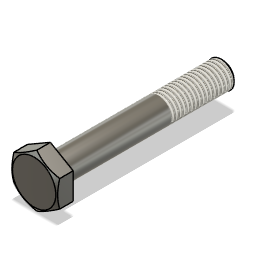
body part (v2~recovered) (Autodesk Fusion 360 archive; units mm, degrees)
design "Heavy Hex Screw ANSI B18.2.3.3M - M14x2 x 90 Steel Grade 2 Plain"
description: Heavy Hex Screw ANSI B18.2.3.3M - M14x2 x 90
Autodesk Fusion 360 part; units mm, degrees
sketch "Sketch1" plane through (0, 0, 0) normal (0, 1, 0) x (1, 0, 0)
  line L0 (-7, 0) -> (-7, 90)
  line L1 (-7, 90) -> (0, 90)
  line L2 (0, 90) -> (0, -9.09)
  line L3 (-11.25, -0.6) -> (-13.86, -0.6)
  line L4 (-13.86, -0.6) -> (-13.86, -7.6697)
  line L5 (-11.25, -0.6) -> (-10.9036, 0)
  line L6 (-10.9036, 0) -> (-7, 0)
  line L7 (0, -9.09) -> (-11.4, -9.09)
  line L8 (-13.86, -7.6697) -> (-11.4, -9.09)
  dimension "d81" = 27.72
  dimension "d123" = 0.6
  dimension "d127" = 90
  dimension "d149" = 14
  dimension "d157" = 30
  dimension "d158" = 22.8
  dimension "d162" = 9.09
  dimension "d163" = 30
  dimension "d164" = 22.5
  constraint perpendicular L0 L1
  constraint perpendicular L0 L3
  constraint vertical L0
  constraint vertical L2
  constraint parallel L2 L4
  constraint coincident L2 L7.start
  constraint perpendicular L0 L6
  constraint coincident origin L6
  constraint coincident L0.end L1.start
  constraint perpendicular L2 L7
  constraint coincident origin L2
  measures "d123" distance of L3 L6
  measures "d127" distance of L1 L6
  measures "d157" angle of L7 L8
  measures "d162" distance of L6 L7
  measures "d163" angle of L4 L5
revolve "Revolve1" add sketch "Sketch1" angle 360 about axis through (0, 0, -90) along (0, 0, 1)
sketch "Sketch8" plane through (0, 0, 0) normal (0, 0, 1) x (1, 0, 0)
  line L0 (-12, -6.9354) -> (-12, 6.9354)
  circle A0 centre (0, 0) radius 10.45
  circle A1 centre (0, 0) radius 13.86
  circle A2 centre (0, 0) radius 13.86
  dimension "d114" = 12
  constraint vertical L0
  constraint coincident L0.end A1
  constraint coincident L0.start A2
  measures "d114" distance of A0.centre L0
extrude "Extrude5" cut sketch "Sketch8" along normal through all contours L0 A1 A2 picked at (-12.3001, -1.6893)
pattern_circular "C-Pattern2" count 6 over 360 about axis through (0, 0, 1.75) along (0, 0, 1) of "Extrude5"
thread "Thread2" "ISO Metric profile 14.0 M14x2 6g" major diameter 13.822 minor diameter 11.534 pitch 2 angle 60 resizes the face on face at (-6.9652, 0.697, -60) from (0, 0, -56) to (0, 0, -90)
fillet "Fillet6" radius 0.6 1 edges at (6.911, 0, 0)
sketch "Sketch15" plane through (0, 0, 0) normal (0, 1, 0) x (1, 0, 0)
  line L0 (-7.14, 90) -> (-7.14, 88.7731)
  line L1 (-7.14, 88.7731) -> (-5.7731, 90)
  line L2 (0, 90) -> (0, -9.09)
  line L3 (-7.14, 90) -> (0, 90)
  dimension "d152" = 7.14
  dimension "d153" = 5.7731
  dimension "d154" = 1.2269
  constraint coincident L2.start L3.end
  constraint perpendicular L2 L3
  constraint coincident L1.end L3
  constraint perpendicular L0 L3
  measures "d152" horizontal distance of origin L0.start
  measures "d153" horizontal distance of origin L1.end
  measures "d154" distance of L0.start L0.end
revolve "Revolve4" cut sketch "Sketch15" angle 360 about axis through (0, 0, 1.75) along (0, 0, 1)
equation "adsk_nomlen = 90.00 mm"
equation "adsk_headh = 9.09 mm"
equation "adsk_headdia = 27.72 mm"
equation "adsk_nomdia = 14.00 mm"
equation "d81 = adsk_headdia"
equation "adsk_waflat = 24.00 mm"
equation "d114 = adsk_waflat / 2"
equation "adsk_thrlen = 34.00 mm"
equation "adsk_chamang2 = 30.00 deg"
equation "adsk_midfillet = 0.60 mm"
equation "d123 = adsk_necklen"
equation "adsk_necklen = 0.60 mm"
equation "adsk_neckdia = 22.50 mm"
equation "d127 = adsk_nomlen"
equation "d138 = adsk_midfillet"
equation "d140 = min(adsk_thrlen; adsk_nomlen - adsk_midfillet - 0.01 mm)"
equation "adsk_endpointdia = 11.5462 mm"
equation "adsk_startlen = 1.2269 mm"
equation "d149 = adsk_nomdia"
equation "d152 = adsk_nomdia * 0.51"
equation "d153 = adsk_endpointdia / 2"
equation "d154 = adsk_startlen"
equation "d157 = adsk_chamang2"
equation "d158 = adsk_waflat * 0.95"
equation "adsk_neckang = 30 deg"
equation "d162 = adsk_headh"
equation "d163 = adsk_neckang"
equation "d164 = adsk_neckdia"

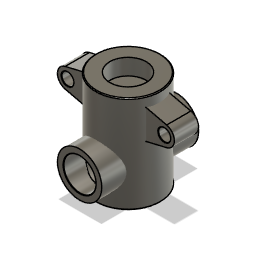
design "wheel hub"
Autodesk Fusion 360 part; units mm, degrees
sketch "Sketch1" plane through (0, 0, 0) normal (0, 0, 1) x (1, 0, 0)
  line L0 (0, 0) -> (40, 0)
  line L1 (40, 0) -> (40, 120)
  line L2 (40, 120) -> (0, 120)
  line L3 (0, 120) -> (0, 0)
  dimension "d1" = 40
  dimension "d2" = 120
  constraint horizontal L0
  constraint vertical L1
  constraint horizontal L2
  constraint vertical L3
  constraint coincident L0.start L3.end
  measures "d1" distance of L1.end L2.end
  measures "d2" distance of L0.end L1.end
revolve "Revolve1" add sketch "Sketch1" angle 360 about axis through (0, 120, 0) along (0, -1, 0) makes body 1
sketch "Sketch2" plane through (0, 0, 0) normal (0, 0, 1) x (1, 0, 0)
sketch "Sketch3" plane through (0, 0, 0) normal (0, 0, 1) x (1, 0, 0)
  line L0 (0, 150) -> (0, -10) construction
  line L1 (-70, 90) -> (60, 90) construction
  line L2 (30, 110) -> (30, 70)
  line L3 (30, 70) -> (62.898, 77.8406)
  line L4 (30, 110) -> (62.898, 102.1594)
  circle A0 centre (60, 90) radius 7.5
  arc A1 (62.898, 77.8406) -> (62.898, 102.1594) centre (60, 90) ccw
  point P0 (40, 120)
  dimension "d4" = 25
  dimension "d5" = 20
  dimension "d6" = 40
  dimension "d7" = 10
  dimension "d8" = 15
  constraint vertical L0
  constraint perpendicular L0 L1
  constraint coincident L1.end A0.centre
  constraint perpendicular L1 L2
  constraint tangent L4 A1
  constraint tangent L3 A1
  constraint concentric A0 A1
  measures "d4" diameter of A1
  measures "d5" distance of L1 L2.start
  measures "d6" distance of L2.start L2.end
  measures "d7" horizontal distance of L2.start P0
  measures "d8" diameter of A0
extrude "Extrude1" add sketch "Sketch3" along normal blind 15 and the other way blind 15 separate body makes body 2
sketch "Sketch4" plane through (0, 0, 0) normal (0, 0, 1) x (1, 0, 0)
mirror "Mirror1" about plane through (0, 0, 0) normal (1, 0, 0) of bodies 2 makes body 3
sketch "Sketch5" plane through (0, 0, 0) normal (0, 0, 1) x (1, 0, 0)
  circle A0 centre (0, 40) radius 27.5
  line L0 (-40, 0) -> (40, 0)
  dimension "d15" = 55
  dimension "d16" = 40
  measures "d15" diameter of A0
  measures "d16" distance of A0.centre L0
extrude "Extrude2" add sketch "Sketch5" along normal blind 60 and the other way blind 60 separate body makes body 4
sketch "Sketch6" plane through (0, 0, 60) normal (0, 0, 1) x (1, 0, 0)
  circle A0 centre (0, 40) radius 27.5
  circle A1 centre (0, 40) radius 20
  dimension "d21" = 40
  constraint concentric A0 A1
  measures "d21" diameter of A1
extrude "Extrude3" cut sketch "Sketch6" along normal blind 60 and the other way blind 60 contours A1 bodies 1 4
sketch "Sketch7" plane through (0, 120, 0) normal (0, 1, 0) x (-1, 0, 0)
  circle A0 centre (0, 0) radius 40
  circle A1 centre (0, 0) radius 22.5
  dimension "d26" = 45
  constraint concentric A0 A1
  measures "d26" diameter of A1
extrude "Extrude4" cut 4 faces at (-6.8687, 44.386, 0) (-6.8687, 44.386, 0) (-6.8687, 44.386, 0) (-6.8687, 44.386, 0) along direction (0, 0, 1) blind 60 and the other way blind 60 on bodies 1 4 bodies 1 4
extrude "Extrude5" cut sketch "Sketch7" along normal blind 0 and the other way blind 20 contours A1 bodies 1
fillet "Fillet1" radius 1 12 edges at (20, 40, 34.641) (20, 40, -34.641) (-37.2931, 0, -14.4646) (-37.2931, 120, -14.4646) (30, 90, 15) (30, 110, 0) (30, 90, -15) (30, 70, 0) (-30, 90, 15) (-30, 110, 0) (-30, 90, -15) (-30, 70, 0) 1 faces at (23.3497, 53.3659, 32.4776) on bodies 1 2 3
chamfer "Chamfer1" distance 0.5 angle 45 6 edges at (53.0075, 92.7121, 15) (53.0075, 87.2879, -15) (-53.0075, 92.7121, 15) (-53.0075, 87.2879, -15) (-18.6465, 47.2323, 60) (-18.6465, 32.7677, -60) measured on face at (38.3212, 90, 15) measured on face at (38.3212, 90, -15) measured on face at (-67.4627, 89.2532, 5) measured on face at (-67.4627, 89.2532, 5) measured on face at (24.8232, 37.6402, 60) measured on face at (24.8232, 37.6402, -60) on bodies 2 3 4

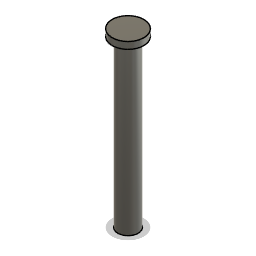
design "landing gear piston"
Autodesk Fusion 360 part; units mm, degrees
sketch "Sketch1" plane through (0, 0, 0) normal (0, 0, 1) x (1, 0, 0)
  line L0 (0, 0) -> (0, 380)
  line L1 (0, 380) -> (35, 380)
  line L2 (35, 380) -> (35, 365)
  line L3 (35, 365) -> (22.5, 365)
  line L4 (22.5, 365) -> (22.5, 0)
  line L5 (22.5, 0) -> (0, 0)
  dimension "d2" = 380
  dimension "d3" = 22.5
  dimension "d4" = 35
  dimension "d5" = 15
  constraint coincident L0.start L5.end
  constraint perpendicular L1 L2
  constraint perpendicular L3 L4
  constraint perpendicular L0 L5
  measures "d2" distance of L0.start L0.end
  measures "d3" distance of L4.end L0.start
  measures "d4" distance of L0.end L1.end
  measures "d5" distance of L1.end L2.end
revolve "Revolve1" add sketch "Sketch1" angle 360 about axis through (0, 0, 0) along (0, 1, 0)

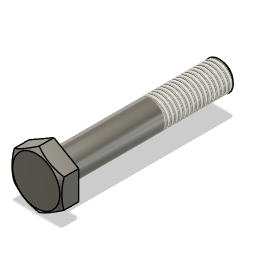
design "Heavy Hex Screw ANSI B18.2.3.3M - M14x2 x 80 Steel Grade 2 Plain"
description: Heavy Hex Screw ANSI B18.2.3.3M - M14x2 x 80
Autodesk Fusion 360 part; units mm, degrees
sketch "Sketch1" plane through (0, 0, 0) normal (0, 1, 0) x (1, 0, 0)
  line L0 (-7, 0) -> (-7, 80)
  line L1 (-7, 80) -> (0, 80)
  line L2 (0, 80) -> (0, -9.09)
  line L3 (-11.25, -0.6) -> (-13.86, -0.6)
  line L4 (-13.86, -0.6) -> (-13.86, -7.6697)
  line L5 (-11.25, -0.6) -> (-10.9036, 0)
  line L6 (-10.9036, 0) -> (-7, 0)
  line L7 (0, -9.09) -> (-11.4, -9.09)
  line L8 (-13.86, -7.6697) -> (-11.4, -9.09)
  dimension "d81" = 27.72
  dimension "d123" = 0.6
  dimension "d127" = 80
  dimension "d149" = 14
  dimension "d157" = 30
  dimension "d158" = 22.8
  dimension "d162" = 9.09
  dimension "d163" = 30
  dimension "d164" = 22.5
  constraint perpendicular L0 L1
  constraint perpendicular L0 L3
  constraint vertical L0
  constraint vertical L2
  constraint parallel L2 L4
  constraint coincident L2 L7.start
  constraint perpendicular L0 L6
  constraint coincident origin L6
  constraint coincident L0.end L1.start
  constraint perpendicular L2 L7
  constraint coincident origin L2
  measures "d123" distance of L3 L6
  measures "d127" distance of L1 L6
  measures "d157" angle of L7 L8
  measures "d162" distance of L6 L7
  measures "d163" angle of L4 L5
revolve "Revolve1" add sketch "Sketch1" angle 360 about axis through (0, 0, -80) along (0, 0, 1)
sketch "Sketch8" plane through (0, 0, 0) normal (0, 0, 1) x (1, 0, 0)
  line L0 (-12, -6.9354) -> (-12, 6.9354)
  circle A0 centre (0, 0) radius 10.45
  circle A1 centre (0, 0) radius 13.86
  circle A2 centre (0, 0) radius 13.86
  dimension "d114" = 12
  constraint vertical L0
  constraint coincident L0.end A1
  constraint coincident L0.start A2
  measures "d114" distance of A0.centre L0
extrude "Extrude5" cut sketch "Sketch8" along normal through all contours L0 A1 A2 picked at (-12.3001, -1.6893)
pattern_circular "C-Pattern2" count 6 over 360 about axis through (0, 0, 1.75) along (0, 0, 1) of "Extrude5"
thread "Thread2" "ISO Metric profile 14.0 M14x2 6g" major diameter 13.822 minor diameter 11.534 pitch 2 angle 60 resizes the face on face at (-6.9913, 0.3489, -53.3333) from (0, 0, -46) to (0, 0, -80)
fillet "Fillet6" radius 0.6 1 edges at (6.911, 0, 0)
sketch "Sketch15" plane through (0, 0, 0) normal (0, 1, 0) x (1, 0, 0)
  line L0 (-7.14, 80) -> (-7.14, 78.7731)
  line L1 (-7.14, 78.7731) -> (-5.7731, 80)
  line L2 (0, 80) -> (0, -9.09)
  line L3 (-7.14, 80) -> (0, 80)
  dimension "d152" = 7.14
  dimension "d153" = 5.7731
  dimension "d154" = 1.2269
  constraint coincident L2.start L3.end
  constraint perpendicular L2 L3
  constraint coincident L1.end L3
  constraint perpendicular L0 L3
  measures "d152" horizontal distance of origin L0.start
  measures "d153" horizontal distance of origin L1.end
  measures "d154" distance of L0.start L0.end
revolve "Revolve4" cut sketch "Sketch15" angle 360 about axis through (0, 0, 1.75) along (0, 0, 1)
equation "adsk_nomlen = 80.00 mm"
equation "adsk_headh = 9.09 mm"
equation "adsk_headdia = 27.72 mm"
equation "adsk_nomdia = 14.00 mm"
equation "d81 = adsk_headdia"
equation "adsk_waflat = 24.00 mm"
equation "d114 = adsk_waflat / 2"
equation "adsk_thrlen = 34.00 mm"
equation "adsk_chamang2 = 30.00 deg"
equation "adsk_midfillet = 0.60 mm"
equation "d123 = adsk_necklen"
equation "adsk_necklen = 0.60 mm"
equation "adsk_neckdia = 22.50 mm"
equation "d127 = adsk_nomlen"
equation "d138 = adsk_midfillet"
equation "d140 = min(adsk_thrlen; adsk_nomlen - adsk_midfillet - 0.01 mm)"
equation "adsk_endpointdia = 11.5462 mm"
equation "adsk_startlen = 1.2269 mm"
equation "d149 = adsk_nomdia"
equation "d152 = adsk_nomdia * 0.51"
equation "d153 = adsk_endpointdia / 2"
equation "d154 = adsk_startlen"
equation "d157 = adsk_chamang2"
equation "d158 = adsk_waflat * 0.95"
equation "adsk_neckang = 30 deg"
equation "d162 = adsk_headh"
equation "d163 = adsk_neckang"
equation "d164 = adsk_neckdia"

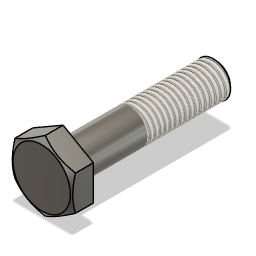
design "Heavy Hex Screw ANSI B18.2.3.3M - M14x2 x 60 Steel Grade 2 Plain"
description: Heavy Hex Screw ANSI B18.2.3.3M - M14x2 x 60
Autodesk Fusion 360 part; units mm, degrees
sketch "Sketch1" plane through (0, 0, 0) normal (0, 1, 0) x (1, 0, 0)
  line L0 (-7, 0) -> (-7, 60)
  line L1 (-7, 60) -> (0, 60)
  line L2 (0, 60) -> (0, -9.09)
  line L3 (-11.25, -0.6) -> (-13.86, -0.6)
  line L4 (-13.86, -0.6) -> (-13.86, -7.6697)
  line L5 (-11.25, -0.6) -> (-10.9036, 0)
  line L6 (-10.9036, 0) -> (-7, 0)
  line L7 (0, -9.09) -> (-11.4, -9.09)
  line L8 (-13.86, -7.6697) -> (-11.4, -9.09)
  dimension "d81" = 27.72
  dimension "d123" = 0.6
  dimension "d127" = 60
  dimension "d149" = 14
  dimension "d157" = 30
  dimension "d158" = 22.8
  dimension "d162" = 9.09
  dimension "d163" = 30
  dimension "d164" = 22.5
  constraint perpendicular L0 L1
  constraint perpendicular L0 L3
  constraint vertical L0
  constraint vertical L2
  constraint parallel L2 L4
  constraint coincident L2 L7.start
  constraint perpendicular L0 L6
  constraint coincident origin L6
  constraint coincident L0.end L1.start
  constraint perpendicular L2 L7
  constraint coincident origin L2
  measures "d123" distance of L3 L6
  measures "d127" distance of L1 L6
  measures "d157" angle of L7 L8
  measures "d162" distance of L6 L7
  measures "d163" angle of L4 L5
revolve "Revolve1" add sketch "Sketch1" angle 360 about axis through (0, 0, -60) along (0, 0, 1)
sketch "Sketch8" plane through (0, 0, 0) normal (0, 0, 1) x (1, 0, 0)
  line L0 (-12, -6.9354) -> (-12, 6.9354)
  circle A0 centre (0, 0) radius 10.45
  circle A1 centre (0, 0) radius 13.86
  circle A2 centre (0, 0) radius 13.86
  dimension "d114" = 12
  constraint vertical L0
  constraint coincident L0.end A1
  constraint coincident L0.start A2
  measures "d114" distance of A0.centre L0
extrude "Extrude5" cut sketch "Sketch8" along normal through all contours L0 A1 A2 picked at (-12.3001, -1.6893)
pattern_circular "C-Pattern2" count 6 over 360 about axis through (0, 0, 1.75) along (0, 0, 1) of "Extrude5"
thread "Thread2" "ISO Metric profile 14.0 M14x2 6g" major diameter 13.822 minor diameter 11.534 pitch 2 angle 60 resizes the face on face at (-6.9652, 0.697, -40) from (0, 0, -26) to (0, 0, -60)
fillet "Fillet6" radius 0.6 1 edges at (6.911, 0, 0)
sketch "Sketch15" plane through (0, 0, 0) normal (0, 1, 0) x (1, 0, 0)
  line L0 (-7.14, 60) -> (-7.14, 58.7731)
  line L1 (-7.14, 58.7731) -> (-5.7731, 60)
  line L2 (0, 60) -> (0, -9.09)
  line L3 (-7.14, 60) -> (0, 60)
  dimension "d152" = 7.14
  dimension "d153" = 5.7731
  dimension "d154" = 1.2269
  constraint coincident L2.start L3.end
  constraint perpendicular L2 L3
  constraint coincident L1.end L3
  constraint perpendicular L0 L3
  measures "d152" horizontal distance of origin L0.start
  measures "d153" horizontal distance of origin L1.end
  measures "d154" distance of L0.start L0.end
revolve "Revolve4" cut sketch "Sketch15" angle 360 about axis through (0, 0, 1.75) along (0, 0, 1)
equation "adsk_nomlen = 60.00 mm"
equation "adsk_headh = 9.09 mm"
equation "adsk_headdia = 27.72 mm"
equation "adsk_nomdia = 14.00 mm"
equation "d81 = adsk_headdia"
equation "adsk_waflat = 24.00 mm"
equation "d114 = adsk_waflat / 2"
equation "adsk_thrlen = 34.00 mm"
equation "adsk_chamang2 = 30.00 deg"
equation "adsk_midfillet = 0.60 mm"
equation "d123 = adsk_necklen"
equation "adsk_necklen = 0.60 mm"
equation "adsk_neckdia = 22.50 mm"
equation "d127 = adsk_nomlen"
equation "d138 = adsk_midfillet"
equation "d140 = min(adsk_thrlen; adsk_nomlen - adsk_midfillet - 0.01 mm)"
equation "adsk_endpointdia = 11.5462 mm"
equation "adsk_startlen = 1.2269 mm"
equation "d149 = adsk_nomdia"
equation "d152 = adsk_nomdia * 0.51"
equation "d153 = adsk_endpointdia / 2"
equation "d154 = adsk_startlen"
equation "d157 = adsk_chamang2"
equation "d158 = adsk_waflat * 0.95"
equation "adsk_neckang = 30 deg"
equation "d162 = adsk_headh"
equation "d163 = adsk_neckang"
equation "d164 = adsk_neckdia"

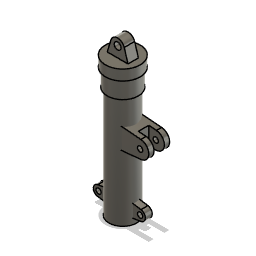
design "strut"
Autodesk Fusion 360 part; units mm, degrees
sketch "Sketch1" plane through (0, 0, 0) normal (0, 0, 1) x (1, 0, 0)
  line L0 (0, 120) -> (0, -70) construction
  line L1 (-120, 5) -> (170, 5) construction
  line L2 (0, 405) -> (50, 405)
  line L3 (50, 405) -> (50, 375)
  line L4 (45, 375) -> (45, 325)
  line L5 (45, 375) -> (50, 375)
  line L6 (45, 325) -> (40, 325)
  line L7 (40, 325) -> (40, 5)
  line L8 (22.5, 5) -> (22.5, 10)
  line L9 (22.5, 10) -> (35, 10)
  line L10 (35, 10) -> (35, 390)
  line L11 (35, 390) -> (0, 390)
  line L12 (0, 405) -> (0, 390)
  line L13 (22.5, 5) -> (40, 5)
  dimension "d1" = 400
  dimension "d2" = 50
  dimension "d5" = 5
  dimension "d6" = 5
  dimension "d8" = 30
  dimension "d9" = 80
  dimension "d10" = 15
  dimension "d11" = 40
  dimension "d12" = 35
  dimension "d13" = 5
  dimension "d14" = 22.5
  constraint horizontal L1
  constraint coincident L0 L2.start
  constraint perpendicular L0 L2
  constraint perpendicular L2 L3
  constraint coincident L1 L8.start
  constraint coincident L0 L11.end
  constraint perpendicular L0 L11
  constraint perpendicular L7 L13
  measures "d1" distance of L1 L2
  measures "d2" distance of L2.start L2.end
  measures "d5" distance of L3.end L4.start
  measures "d6" distance of L4.end L6.end
  measures "d8" distance of L2 L5
  measures "d9" distance of L2 L6
  measures "d10" distance of L2 L11
  measures "d11" distance of L7 L12
  measures "d12" distance of L10 L12
  measures "d13" distance of L8.start L8.end
  measures "d14" distance of L0 L8
revolve "Revolve1" add sketch "Sketch1" angle 360 about axis through (0, 120, 0) along (0, -1, 0) makes body 1
sketch "Sketch2" plane through (0, 0, 0) normal (0, 0, 1) x (1, 0, 0)
  line L0 (-80, 405) -> (80, 405) construction
  line L1 (-20, 405) -> (20, 405)
  line L2 (0, 435) -> (0, 324.2267) construction
  line L3 (-25, 405) -> (25, 405)
  line L4 (-30, 405) -> (30, 405)
  line L5 (-30, 405) -> (-19.1389, 440.8055)
  line L6 (30, 405) -> (19.1389, 440.8055)
  circle A0 centre (0, 435) radius 10
  arc A1 (19.1389, 440.8055) -> (-19.1389, 440.8055) centre (0, 435) ccw
  dimension "d18" = 60
  dimension "d19" = 30
  dimension "d20" = 40
  dimension "d21" = 30
  dimension "d22" = 20
  constraint horizontal L0
  constraint coincident L0 L1.start
  constraint coincident L0 L1.end
  constraint vertical L2
  constraint coincident L0 L3.start
  constraint coincident L0 L3.end
  constraint perpendicular L2 L3
  constraint coincident L0 L4.end
  constraint parallel L0 L4
  constraint coincident L2.start A0.centre
  constraint tangent L5 A1
  constraint tangent L6 A1
  measures "d18" distance of L4.start L4.end
  measures "d19" distance of L2 L4.start
  measures "d20" diameter of A1
  measures "d21" distance of L3 L2.start
  measures "d22" diameter of A0
extrude "Extrude1" add sketch "Sketch2" along normal blind 15 and the other way blind 15 bodies 1
sketch "Sketch3" plane through (0, 0, 0) normal (0, 0, 1) x (1, 0, 0)
  line L0 (0, -15) -> (0, 100) construction
  line L1 (-100, 40) -> (100, 40) construction
  line L2 (-40, 5) -> (40, 5) construction
  line L3 (30, 60) -> (30, 20)
  line L4 (30, 60) -> (62.374, 54.811)
  line L5 (30, 20) -> (62.374, 25.189)
  circle A0 centre (60, 40) radius 7.5
  arc A1 (62.374, 25.189) -> (62.374, 54.811) centre (60, 40) ccw
  dimension "d27" = 35
  dimension "d29" = 40
  dimension "d30" = 20
  dimension "d31" = 30
  dimension "d32" = 30
  dimension "d33" = 30
  dimension "d34" = 15
  constraint vertical L0
  constraint horizontal L1
  constraint perpendicular L1 L3
  constraint coincident L1 A0.centre
  constraint tangent L4 A1
  constraint tangent L5 A1
  constraint concentric A0 A1
  measures "d27" distance of L1 L2
  measures "d29" distance of L3.start L3.end
  measures "d30" distance of L1 L3.start
  measures "d31" distance of L0 L3
  measures "d32" diameter of A1
  measures "d33" horizontal distance of L3.start A0.centre
  measures "d34" diameter of A0
extrude "Extrude2" add sketch "Sketch3" along normal blind 10 and the other way blind 10 separate body makes body 2
mirror "Mirror1" about plane through (0, 0, 0) normal (1, 0, 0) of "Extrude2" makes body 3
sketch "Sketch4" plane through (0, 0, 0) normal (0, 0, 1) x (1, 0, 0)
  line L0 (0, 200) -> (0, 210) construction
  line L1 (0, 210) -> (0, 380) construction
  line L2 (-150, 225) -> (150, 225) construction
  line L3 (-45, 325) -> (45, 325) construction
  line L4 (20, 255) -> (20, 195)
  line L5 (20, 255) -> (82.0416, 249.9165)
  line L6 (20, 195) -> (32.5622, 195)
  line L7 (32.5622, 195) -> (82.5524, 200.1306)
  circle A0 centre (80, 225) radius 7.5
  arc A1 (82.5524, 200.1306) -> (82.0416, 249.9165) centre (80, 225) ccw
  dimension "d41" = 100
  dimension "d42" = 50
  dimension "d43" = 60
  dimension "d44" = 30
  dimension "d45" = 60
  dimension "d46" = 15
  constraint vertical L0
  constraint parallel L0 L1
  constraint perpendicular L1 L2
  constraint coincident L2 A0.centre
  constraint perpendicular L2 L4
  constraint perpendicular L4 L6
  constraint tangent L7 A1
  constraint tangent L5 A1
  constraint concentric A0 A1
  measures "d41" distance of L2 L3
  measures "d42" diameter of A1
  measures "d43" distance of L4.start L4.end
  measures "d44" distance of L2 L4.start
  measures "d45" distance of A0.centre L4
  measures "d46" diameter of A0
extrude "Extrude3" add sketch "Sketch4" along normal blind 30 and the other way blind 30 separate body makes body 4
sketch "Sketch5" plane through (0, 0, 0) normal (0, 0, 1) x (1, 0, 0)
  line L0 (60, 265) -> (130, 265)
  line L1 (130, 265) -> (130, 185)
  line L2 (130, 185) -> (60, 185)
  line L3 (60, 185) -> (60, 265)
  circle A0 centre (80, 225) radius 7.5
  dimension "d51" = 80
  dimension "d52" = 70
  dimension "d53" = 40
  dimension "d54" = 20
  constraint horizontal L0
  constraint vertical L1
  constraint horizontal L2
  constraint vertical L3
  measures "d51" distance of L0.end L1.end
  measures "d52" distance of L0.start L0.end
  measures "d53" distance of L0 A0.centre
  measures "d54" distance of L3 A0.centre
extrude "Extrude4" cut sketch "Sketch5" along normal blind 15 and the other way blind 15 bodies 4
